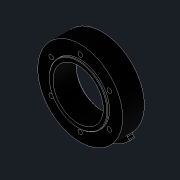
# Autodesk Inventor part: unit-base7
Saved by Autodesk Inventor 2022 (Build 260153000, 153)
## iProperties
Created: 2021-07-16
Part Number: unit-base7
Material: ABS プラスチック
Document SubType Name: Modeling
Designer: yuta0
Density: 1.06 g/cm^3
Appearance: 滑らか - 黒
Mass: 62.9705 g
Surface Area: 165.869 cm^2
Volume: 59.4061 cm^3
購入先: 印刷
在庫数: 0.0
Author: yuta0
Autodesk Inventor part; units mm, degrees
ref_plane "YZ Plane" through (0, 0, 0) normal (1, 0, 0) x (0, 1, 0)
ref_plane "XZ Plane" through (0, 0, 0) normal (0, 1, 0) x (-1, 0, 0)
ref_plane "XY Plane" through (0, 0, 0) normal (0, 0, 1) x (1, 0, 0)
sketch "スケッチ1" plane through (0, 0, 0) normal (1, 0, 0) x (0, 1, 0)
  line L0 (40.5, 0) -> (24, 0)
  line L1 (24, 0) -> (24, -20.7)
  line L2 (24, -20.7) -> (40.5, -20.7)
  line L3 (40.5, -20.7) -> (40.5, 0)
  line L4 (0, -24.84) -> (0, 4.14) projected
  point P0 (0, 0)
  dimension "d0" = 24
  dimension "d2" = 40.5
  dimension "d3" = 20.7
  constraints: 8 end point, 2 parallel, 1 horizontal, 1 horizontal alignment, 1 perpendicular
  measures "d0" distance from line of point (0, 0) L1
  measures "d2" distance from line of point (0, 0) L3
  measures "d3" distance of L2.end L0.start
revolve "回転1" add sketch "スケッチ1" angle 360 about axis through (0, 0, -10) along (0, 0, 1)
sketch "スケッチ2" plane through (0, 0, 0) normal (0, 0, 1) x (1, 0, 0)
  circle A0 centre (0, 0) radius 32
  point P0 (0, 32)
  point P1 (-27.7128, 16)
  point P2 (-27.7128, -16)
  point P3 (0, -32)
  point P4 (27.7128, -16)
  point P5 (27.7128, 16)
  dimension "d5" = 64
  dimension "d8" = 360
  constraints: 1 coincident, 1 vertical alignment, 9 other
hole "穴1" at (0, 32, 0) at (-27.7128, 16, 0) at (-27.7128, -16, 0) at (0, -32, 0) at (27.7128, -16, 0) at (27.7128, 16, 0) direction (0, 0, -1) diameter 4.3 end through all clearance for "Socket Head Cap Screw" size "M4" standard "Ansi Metric M Profile"
sketch "スケッチ3" plane through (0, 0, -20.7) normal (0, 0, 1) x (1, 0, 0)
  circle A0 centre (0, 0) radius 40.5 projected
  circle A1 centre (0, 0) radius 44.5
  line L0 (0, 0) -> (-31.4663, -31.4663)
  line L1 (0, 0) -> (31.4663, -31.4663)
  line L2 (0, 62.3) -> (0, -62.3) projected
  point P0 (-28.6378, -28.6378)
  point P1 (28.6378, -28.6378)
  point P2 (19.901, -39.802)
  dimension "d17" = 4
  dimension "d23" = 45
  dimension "d24" = 45
  constraints: 4 end point, 2 point on circle, 1 centre point
  measures "d17" radial gap between concentric circles of A0 A1
  measures "d23" angle of L2 L1
  measures "d24" angle of L0 L2
extrude "押し出し1" add sketch "スケッチ3" along normal blind 5 contours L1 A1 L2 A0 | A0 L2 A1 L0 picked at (28.2757, -32.3682) picked at (-28.2757, -32.3682)
fillet "フィレット1" radius 1 4 edges at (-31.4663, -31.4663, -18.2) (31.4663, -31.4663, -18.2) (28.6378, -28.6378, -18.2) (-28.6378, -28.6378, -18.2)
sketch "スケッチ5" plane through (0, 0, 0) normal (0, 0, 1) x (1, 0, 0)
  circle A0 centre (0, 0) radius 24 projected
  circle A1 centre (0, 0) radius 28
  dimension "d28" = 4
  constraints: 1 centre point
  measures "d28" radial gap between concentric circles of A0 A1
extrude "押し出し3" add sketch "スケッチ5" along normal blind 2
chamfer "面取り1" distance 0.5 angle 45 1 edges at (-28, 0, 2)
chamfer "面取り2" distance 0.5 angle 45 1 edges at (0, -24, -20.7)
